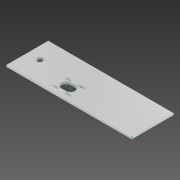
# Autodesk Inventor part: bovenarm - links
Saved by Autodesk Inventor 2020 (Build 240168000, 168)
## iProperties
Created: 2020-05-18
Part Number: bovenarm - links
Material: Generic
Document SubType Name: Modeling
Designer: stefa
Density: 1 g/cm^3
Appearance: Aluminum - Polished
Author: stefa
Autodesk Inventor part; units mm, degrees
ref_plane "YZ Plane" through (0, 0, 0) normal (1, 0, 0) x (0, 1, 0)
ref_plane "XZ Plane" through (0, 0, 0) normal (0, 1, 0) x (-1, 0, 0)
ref_plane "XY Plane" through (0, 0, 0) normal (0, 0, 1) x (1, 0, 0)
sketch "Sketch1" plane through (0, 0, 0) normal (0, 1, 0) x (-1, 0, 0)
  line L0 (0, 0) -> (300, 0)
  line L1 (300, 0) -> (300, -100)
  line L2 (300, -100) -> (0, -100)
  line L3 (0, -100) -> (0, 0)
  circle A0 centre (270, -50) radius 6
  line L4 (185.2943, -28) -> (175.2943, -28) construction
  line L5 (185.2943, -16.9) -> (175.2943, -16.9)
  line L6 (175.2943, -39.1) -> (185.2943, -39.1)
  arc A1 (185.2943, -39.1) -> (185.2943, -16.9) centre (185.2943, -28) ccw
  arc A2 (175.2943, -16.9) -> (175.2943, -39.1) centre (175.2943, -28) ccw
  line L7 (200.7943, -43.5) -> (190.7943, -43.5) construction
  line L8 (200.7943, -42.2) -> (190.7943, -42.2)
  line L9 (190.7943, -44.8) -> (200.7943, -44.8)
  arc A3 (200.7943, -44.8) -> (200.7943, -42.2) centre (200.7943, -43.5) ccw
  arc A4 (190.7943, -42.2) -> (190.7943, -44.8) centre (190.7943, -43.5) ccw
  line L10 (159.7943, -44.8) -> (169.7943, -44.8)
  arc A5 (169.7943, -44.8) -> (169.7943, -42.2) centre (169.7943, -43.5) ccw
  line L11 (169.7943, -43.5) -> (159.7943, -43.5) construction
  line L12 (169.7943, -42.2) -> (159.7943, -42.2)
  arc A6 (159.7943, -42.2) -> (159.7943, -44.8) centre (159.7943, -43.5) ccw
  line L13 (190.7943, -13.8) -> (200.7943, -13.8)
  arc A7 (200.7943, -13.8) -> (200.7943, -11.2) centre (200.7943, -12.5) ccw
  line L14 (200.7943, -12.5) -> (190.7943, -12.5) construction
  line L15 (200.7943, -11.2) -> (190.7943, -11.2)
  arc A8 (190.7943, -11.2) -> (190.7943, -13.8) centre (190.7943, -12.5) ccw
  line L16 (159.7943, -13.8) -> (169.7943, -13.8)
  arc A9 (169.7943, -13.8) -> (169.7943, -11.2) centre (169.7943, -12.5) ccw
  line L17 (169.7943, -12.5) -> (159.7943, -12.5) construction
  line L18 (169.7943, -11.2) -> (159.7943, -11.2)
  arc A10 (159.7943, -11.2) -> (159.7943, -13.8) centre (159.7943, -12.5) ccw
  point P0 (180.2943, -28)
  point P1 (195.7943, -43.5)
  point P2 (164.7943, -43.5)
  point P3 (195.7943, -12.5)
  point P4 (164.7943, -12.5)
  dimension "d0" = 300
  dimension "d1" = 100
  dimension "d16" = 12
  dimension "d18" = 50
  dimension "d24" = 22.2
  dimension "d25" = 2.6
  dimension "d26" = 10
  dimension "d27" = 10
  dimension "d28" = 92.364
  dimension "d29" = 28
  dimension "d30" = 30
  dimension "d31" = 15.5
  dimension "d32" = 15.5
  dimension "d35" = 31
  dimension "d38" = 31
  constraints: 48 end point, 20 point on circle, 11 centre point, 8 tangent, 5 parallel, 3 horizontal, 2 midpoint, 1 perpendicular, 1 vertical, 36 other
  measures "d0" distance of L1.end L2.end
  measures "d1" distance of L0.end L1.end
  measures "d16" diameter of A0
  measures "d18" distance from line of L0 A0.centre
  measures "d24" diameter of A2
  measures "d25" diameter of A4
  measures "d26" distance of L9.start L9.end
  measures "d27" distance of L6.start L6.end
  measures "d28" distance of A0.centre point (180.294, -28)
  measures "d29" distance from line of L0 point (180.294, -28)
  measures "d30" distance from line of L1 A0.centre
  measures "d31" horizontal distance of point (180.294, -28) point (195.794, -43.5)
  measures "d32" horizontal distance of point (195.794, -43.5) point (180.294, -28)
  measures "d35" distance of L9.start L10.start
  measures "d38" distance of L9.start L13.start
extrude "Extrusion1" add sketch "Sketch1" along normal blind 4
sketch "Sketch3" plane through (0, 4, 0) normal (0, 1, 0) x (1, 0, 0)
  line L0 (-196.3943, 28) -> (-164.1943, 28) construction
  arc A0 (-185.2943, 39.1) -> (-185.2943, 16.9) centre (-185.2943, 28) ccw construction
  arc A1 (-175.2943, 16.9) -> (-175.2943, 39.1) centre (-175.2943, 28) ccw construction
  point P0 (0, 0)
  constraints: 2 end point, 2 point on circle, 1 horizontal
equation "\"d18\" = 0.5 * d1"
body "Solid1"
